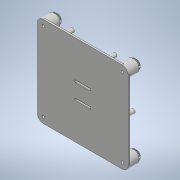
# Autodesk Inventor part: Зажим проводов
Saved by Autodesk Inventor 2020 (Build 240168000, 168)
## iProperties
Created: 2021-04-22
Part Number: Зажим проводов
Material: Типовые
Document SubType Name: Modeling
Designer: I_Love_U_Bogdan
Density: 1 g/cm^3
Appearance: По умолчанию
Author: I_Love_U_Bogdan
Autodesk Inventor part; units mm, degrees
ref_plane "YZ Plane" through (0, 0, 0) normal (1, 0, 0) x (0, 1, 0)
ref_plane "XZ Plane" through (0, 0, 0) normal (0, 1, 0) x (-1, 0, 0)
ref_plane "XY Plane" through (0, 0, 0) normal (0, 0, 1) x (1, 0, 0)
sketch "Эскиз1" plane through (0, 0, 0) normal (0, 0, 1) x (1, 0, 0)
  circle A0 centre (-37.4959, 38.6601) radius 4.5 projected
  circle A1 centre (62.5041, 38.6601) radius 4.5 projected
  line L0 (-47.4959, 36.6601) -> (-44.978, 39.178) projected
  line L1 (-47.4959, 36.6601) -> (-47.4959, -61.7399) projected
  line L2 (-40.4959, -68.7399) -> (-47.4959, -61.7399) projected
  line L3 (-40.4959, -68.7399) -> (65.5041, -68.7399) projected
  line L4 (72.5041, -61.7399) -> (65.5041, -68.7399) projected
  line L5 (72.5041, -61.7399) -> (72.5041, 36.6601) projected
  line L6 (69.9862, 39.178) -> (72.5041, 36.6601) projected
  arc A2 (69.9862, 39.178) -> (56.914, 43.6601) centre (62.5041, 38.6601) ccw projected
  line L7 (56.914, 43.6601) -> (-31.9057, 43.6601) projected
  arc A3 (-31.9057, 43.6601) -> (-44.978, 39.178) centre (-37.4959, 38.6601) ccw projected
  circle A4 centre (-37.4959, -60.7399) radius 4.5 projected
  circle A5 centre (62.5041, -60.7399) radius 4.5 projected
  circle A6 centre (7.5041, -49.0399) radius 2.5 projected
  circle A7 centre (31.8041, -37.6685) radius 2.5 projected
  circle A8 centre (16.6041, 13.1315) radius 2.5 projected
  circle A9 centre (-41.4959, 8.9601) radius 2.5 projected
  circle A10 centre (7.5041, 8.9601) radius 2.5 projected
  circle A11 centre (64.8041, 14.4315) radius 2.5 projected
  circle A12 centre (59.7041, -37.6685) radius 2.5 projected
  circle A13 centre (-41.4959, -49.0399) radius 2.5 projected
  circle A14 centre (-37.4959, 38.6601) radius 7.5
  circle A15 centre (62.5041, 38.6601) radius 7.5
  circle A16 centre (62.5041, -60.7399) radius 7.5
  circle A17 centre (-37.4959, -60.7399) radius 7.5
  circle A18 centre (39.5041, 38.6601) radius 2.5
  circle A19 centre (-14.4959, 38.6601) radius 2.5
  circle A20 centre (-14.4959, 13.6601) radius 2.5
  circle A21 centre (39.5041, 13.6601) radius 2.5
  circle A22 centre (-14.4959, -11.3399) radius 2.5
  circle A23 centre (39.5041, -11.3399) radius 2.5
  circle A24 centre (-14.4959, -36.3399) radius 2.5
  circle A25 centre (39.5041, -36.3399) radius 2.5
  circle A26 centre (-14.4959, -61.3399) radius 2.5
  circle A27 centre (39.5041, -61.3399) radius 2.5
  circle A28 centre (62.5041, -11.3399) radius 2.5
  circle A29 centre (-37.4959, -11.3399) radius 2.5
  point P0 (0, 0)
  dimension "d0" = 3
  dimension "d1" = 3
  dimension "d2" = 3
  dimension "d3" = 3
  dimension "d4" = 5
  dimension "d5" = 5
  dimension "d6" = 23
  dimension "d7" = 23
  dimension "d8" = 5
  dimension "d9" = 5
  dimension "d12" = 25
  dimension "d17" = 5
  dimension "d18" = 5
  dimension "d19" = 0
  dimension "d20" = 50
  dimension "d21" = 50
  constraints: 16 centre point, 1 vertical, 16 other
  measures "d0" radial gap between concentric circles of A0 A14
  measures "d1" radial gap between concentric circles of A1 A15
  measures "d2" radial gap between concentric circles of A5 A16
  measures "d3" radial gap between concentric circles of A4 A17
  measures "d4" diameter of A18
  measures "d5" diameter of A19
  measures "d6" distance of A19.centre A0.centre
  measures "d7" distance of A1.centre A18.centre
  measures "d8" distance from line of L7 A18.centre
  measures "d9" distance from line of L7 A19.centre
  measures "d12" distance of A19.centre A20.centre
  measures "d17" diameter of A28
  measures "d18" diameter of A29
  measures "d19" horizontal distance of A29.centre A4.centre
  measures "d20" vertical distance of A28.centre A18.centre
  measures "d21" vertical distance of A19.centre A29.centre
extrude "Выдавливание1" add sketch "Эскиз1" along normal blind 12 contours A0 | A1 | A3 A14 | A2 A15 | A4 | A5 | A16 | A17 | A18 | A19 | A20 | A21 | A22 | A23 | A24 | A25 | A26 | A27 | A28 | A29
sketch "Эскиз2" plane through (-37.4959, -60.7399, 12) normal (0, 0, 1) x (1, 0, 0)
  circle A0 centre (0, 0) radius 7.5 projected
  circle A1 centre (100, 0) radius 7.5 projected
  circle A2 centre (100, 99.4) radius 7.5 projected
  circle A3 centre (0, 99.4) radius 7.5 projected
  circle A4 centre (0, 0) radius 7.5 projected
  line L0 (0, -7.5) -> (100, -7.5)
  circle A5 centre (100, 0) radius 7.5 projected
  line L1 (107.5, 0) -> (107.5, 99.4)
  circle A6 centre (100, 99.4) radius 7.5 projected
  line L2 (100, 106.9) -> (0, 106.9)
  circle A7 centre (0, 99.4) radius 7.5 projected
  line L3 (-7.5, 99.4) -> (-7.5, 0)
  point P0 (37.4959, 60.7399)
  point P1 (-7.5, 99.4)
  point P2 (0, -7.5)
  point P3 (100, -7.5)
  constraints: 8 end point, 3 horizontal, 3 vertical, 2 vertical alignment, 1 horizontal alignment, 1 perpendicular, 1 point on circle, 1 tangent, 11 other
extrude "Выдавливание2" add sketch "Эскиз2" along normal blind 2
sketch "Эскиз3" plane through (-37.4959, 38.6601, 0) normal (0, 0, -1) x (-1, 0, 0)
  circle A0 centre (-100, 0) radius 4.5 projected
  circle A1 centre (-100, -99.4) radius 4.5 projected
  circle A2 centre (0, -99.4) radius 4.5 projected
  circle A3 centre (0, 0) radius 4.5 projected
  circle A4 centre (0, 0) radius 4.3
  circle A5 centre (-100, 0) radius 4.3
  circle A6 centre (-100, -99.4) radius 4.3
  circle A7 centre (0, -99.4) radius 4.3
  point P0 (-37.4959, -38.6601)
  dimension "d26" = 0.2
  dimension "d27" = 0.2
  dimension "d28" = 0.2
  dimension "d29" = 0.2
  constraints: 4 centre point
  measures "d26" radial gap between concentric circles of A3 A4
  measures "d27" radial gap between concentric circles of A0 A5
  measures "d28" radial gap between concentric circles of A1 A6
  measures "d29" radial gap between concentric circles of A2 A7
extrude "Выдавливание3" add sketch "Эскиз3" along normal blind 2.2 contours A4 | A5 | A6 | A7
sketch "Эскиз4" plane through (-37.4959, 38.6601, -2.2) normal (0, 0, -1) x (-1, 0, 0)
  circle A0 centre (0, 0) radius 4.3 projected
  circle A1 centre (-100, 0) radius 4.3 projected
  circle A2 centre (-100, -99.4) radius 4.3 projected
  circle A3 centre (0, -99.4) radius 4.3 projected
  circle A4 centre (0, 0) radius 6.3
  circle A5 centre (-100, 0) radius 6.3
  circle A6 centre (-100, -99.4) radius 6.3
  circle A7 centre (0, -99.4) radius 6.3
  point P0 (-37.4959, -38.6601)
  dimension "d32" = 2
  dimension "d33" = 2
  dimension "d34" = 2
  dimension "d35" = 2
  constraints: 4 centre point, 1 coincident
  measures "d32" radial gap between concentric circles of A4 A0
  measures "d33" radial gap between concentric circles of A1 A5
  measures "d34" radial gap between concentric circles of A2 A6
  measures "d35" radial gap between concentric circles of A3 A7
extrude "Выдавливание4" add sketch "Эскиз4" along normal blind 2.2 contours A0 | A1 | A2 | A3 | A4 | A5 | A6 | A7
chamfer "Фаска1" distance 2 angle 45 4 edges at (-31.1959, 38.6601, -4.4) (68.8041, 38.6601, -4.4) (68.8041, -60.7399, -4.4) (-31.1959, -60.7399, -4.4)
sketch "Эскиз5" plane through (62.5041, 38.6601, -4.4) normal (0, 0, -1) x (-1, 0, 0)
  circle A0 centre (100, 0) radius 4.3 projected
  circle A1 centre (0, 0) radius 4.3 projected
  circle A2 centre (0, -99.4) radius 4.3 projected
  circle A3 centre (100, -99.4) radius 4.3 projected
  line L0 (101, 10) -> (99, 10)
  line L1 (99, 10) -> (99, -10)
  line L2 (99, -10) -> (101, -10)
  line L3 (101, -10) -> (101, 10)
  line L4 (101, 10) -> (99, -10) construction
  line L5 (99, 10) -> (101, -10) construction
  line L6 (110, 1) -> (90, 1)
  line L7 (90, 1) -> (90, -1)
  line L8 (90, -1) -> (110, -1)
  line L9 (110, -1) -> (110, 1)
  line L10 (110, 1) -> (90, -1) construction
  line L11 (90, 1) -> (110, -1) construction
  arc A4 (-7.5, 0) -> (0, 7.5) centre (0, 0) ccw projected
  line L12 (-7.5, -99.4) -> (-7.5, 0) projected
  arc A5 (0, -106.9) -> (-7.5, -99.4) centre (0, -99.4) ccw projected
  line L13 (100, -106.9) -> (0, -106.9) projected
  arc A6 (107.5, -99.4) -> (100, -106.9) centre (100, -99.4) ccw projected
  line L14 (107.5, 0) -> (107.5, -99.4) projected
  arc A7 (100, 7.5) -> (107.5, 0) centre (100, 0) ccw projected
  line L15 (0, 7.5) -> (100, 7.5) projected
  circle A8 centre (77, -100) radius 2.5 projected
  circle A9 centre (23, -50) radius 2.5 projected
  circle A10 centre (77, -75) radius 2.5 projected
  circle A11 centre (77, -50) radius 2.5 projected
  circle A12 centre (23, 0) radius 2.5 projected
  circle A13 centre (0, -50) radius 2.5 projected
  circle A14 centre (23, -100) radius 2.5 projected
  circle A15 centre (23, -75) radius 2.5 projected
  circle A16 centre (77, 0) radius 2.5 projected
  circle A17 centre (77, -25) radius 2.5 projected
  circle A18 centre (23, -25) radius 2.5 projected
  circle A19 centre (100, -50) radius 2.5 projected
  line L16 (99, -89.4) -> (101, -89.4)
  line L17 (101, -89.4) -> (101, -109.4)
  line L18 (101, -109.4) -> (99, -109.4)
  line L19 (99, -109.4) -> (99, -89.4)
  line L20 (99, -89.4) -> (101, -109.4) construction
  line L21 (101, -89.4) -> (99, -109.4) construction
  line L22 (110, -98.4) -> (90, -98.4)
  line L23 (90, -98.4) -> (90, -100.4)
  line L24 (90, -100.4) -> (110, -100.4)
  line L25 (110, -100.4) -> (110, -98.4)
  line L26 (110, -98.4) -> (90, -100.4) construction
  line L27 (90, -98.4) -> (110, -100.4) construction
  line L28 (-1, -89.4) -> (1, -89.4)
  line L29 (10, -98.4) -> (-10, -98.4)
  line L30 (-10, -98.4) -> (-10, -100.4)
  line L31 (-10, -100.4) -> (10, -100.4)
  line L32 (10, -98.4) -> (-10, -100.4) construction
  line L33 (-10, -98.4) -> (10, -100.4) construction
  line L34 (10, -100.4) -> (10, -98.4)
  line L35 (1, -89.4) -> (1, -109.4)
  line L36 (-1, -89.4) -> (1, -109.4) construction
  line L37 (1, -89.4) -> (-1, -109.4) construction
  line L38 (1, -109.4) -> (-1, -109.4)
  line L39 (-1, -109.4) -> (-1, -89.4)
  line L40 (-1, -10) -> (1, -10)
  line L41 (-10, 1) -> (-10, -1)
  line L42 (10, 1) -> (-10, 1)
  line L43 (-10, -1) -> (10, -1)
  line L44 (10, 1) -> (-10, -1) construction
  line L45 (-10, 1) -> (10, -1) construction
  line L46 (10, -1) -> (10, 1)
  line L47 (1, 10) -> (-1, 10)
  line L48 (1, -10) -> (1, 10)
  line L49 (1, 10) -> (-1, -10) construction
  line L50 (-1, 10) -> (1, -10) construction
  line L51 (-1, 10) -> (-1, -10)
  point P0 (62.5041, -38.6601)
  point P1 (0, -99.4)
  point P2 (0, 0)
  point P3 (1, 1)
  point P4 (-1, 1)
  point P5 (-1, -1)
  point P6 (1, -1)
  point P7 (-1, -98.4)
  point P8 (-1, -100.4)
  point P9 (1, -100.4)
  point P10 (1, -98.4)
  point P11 (99, -100.4)
  point P12 (101, -100.4)
  point P13 (101, -98.4)
  point P14 (99, -98.4)
  point P15 (101, -1)
  point P16 (101, 1)
  point P17 (99, 1)
  point P18 (99, -1)
  dimension "d41" = 2
  dimension "d42" = 20
  dimension "d43" = 20
  dimension "d44" = 2
  dimension "d45" = 2
  dimension "d46" = 20
  dimension "d47" = 20
  dimension "d48" = 2
  dimension "d51" = 100
  constraints: 96 end point, 16 midpoint, 8 parallel, 5 horizontal, 4 perpendicular, 42 other
  measures "d41" distance of L2.end L1.end
  measures "d42" distance of L1.end L0.end
  measures "d43" distance of L8.end L7.end
  measures "d44" distance of L7.end L6.end
  measures "d45" distance of L17.end L18.end
  measures "d46" distance of L16.end L17.end
  measures "d47" distance of L24.end L23.end
  measures "d48" distance of L23.end L22.end
  measures "d51" distance of L16.start L28.start
extrude "Выдавливание5" cut sketch "Эскиз5" against normal blind 5 contours A0 L8 L3 L6 | A0 L6 L9 L8 L14 A7 | L3 L6 L1 A0 | A0 L1 A7 L15 L0 L3 | L3 L8 L1 L6 | L3 A7 L1 A0 | A0 L1 L8 L3 | A7 L14 L8 | L1 L8 A0 L6 | L3 L2 L1 A7 | A0 L8 A7 L6 | L1 L15 A7 | L22 L25 L24 A3 A6 L14 | L14 A6 L22 | A7 L8 L7 L6 | L48 A4 L15 | L15 A4 L48 A1 L51 L47 | L17 A3 L19 A6 | A6 L19 L16 L17 | A3 L24 L17 L22 | L17 L22 L19 A3 | L17 L24 L19 L22 | L42 L46 L43 A4 | A4 L43 A1 L42 | L48 L42 L51 A1 | L17 L18 L19 L13 A6 A3 | A3 L19 L24 L17 | L22 A3 L24 A6 | A6 L24 L23 L22 | L19 L24 A3 L22 | A1 L43 L48 L42 | L48 L43 L51 L42 | L48 L40 L51 A4 | A4 L51 A1 L48 | L42 L51 L43 A1 | A1 L43 A4 L12 L41 L42 | L48 A1 L51 L43 | A6 L13 L19 | L43 L12 A4 | L35 L38 L39 A2 A5 L13 | L13 A5 L35 | L29 A5 L12 | L12 A5 L29 A2 L31 L30 | L31 A2 L29 A5 | A5 L29 L34 L31 | A2 L39 L31 L35 | L31 L35 L29 A2 | L31 L39 L29 L35 | L39 L28 L35 A5 | A5 L35 A2 L39 | L29 L39 L31 A2 | L29 L39 A2 L35
sketch "Эскиз6" plane through (-37.4959, -60.7399, 14) normal (0, 0, 1) x (1, 0, 0)
  arc A0 (107.5, 99.4) -> (100, 106.9) centre (100, 99.4) ccw projected
  arc A1 (100, -7.5) -> (107.5, 0) centre (100, 0) ccw projected
  arc A2 (0, 106.9) -> (-7.5, 99.4) centre (0, 99.4) ccw projected
  arc A3 (-7.5, 0) -> (0, -7.5) centre (0, 0) ccw projected
  circle A4 centre (0, 0) radius 1.5
  circle A5 centre (0, 99.4) radius 1.5
  circle A6 centre (100, 99.4) radius 1.5
  circle A7 centre (100, 0) radius 1.5
  circle A8 centre (77, 49.4) radius 2.5 projected
  circle A9 centre (23, 49.4) radius 2.5 projected
  line L0 (77, 49.4) -> (23, 49.4)
  line L1 (50, 49.4) -> (50, 39.4)
  line L2 (50, 49.4) -> (50, 59.4)
  line L3 (40, 60.4) -> (60, 60.4)
  line L4 (60, 60.4) -> (60, 58.4)
  line L5 (60, 58.4) -> (40, 58.4)
  line L6 (40, 58.4) -> (40, 60.4)
  line L7 (40, 60.4) -> (60, 58.4) construction
  line L8 (60, 60.4) -> (40, 58.4) construction
  line L9 (40, 40.4) -> (60, 40.4)
  line L10 (60, 40.4) -> (60, 38.4)
  line L11 (60, 38.4) -> (40, 38.4)
  line L12 (40, 38.4) -> (40, 40.4)
  line L13 (40, 40.4) -> (60, 38.4) construction
  line L14 (60, 40.4) -> (40, 38.4) construction
  point P0 (37.4959, 60.7399)
  dimension "d58" = 3
  dimension "d59" = 3
  dimension "d60" = 3
  dimension "d61" = 3
  dimension "d64" = 10
  dimension "d65" = 10
  dimension "d66" = 20
  dimension "d67" = 2
  dimension "d68" = 20
  dimension "d69" = 2
  constraints: 30 end point, 5 midpoint, 4 centre point, 4 coincident, 4 parallel, 3 horizontal, 2 perpendicular, 2 vertical
  measures "d58" diameter of A4
  measures "d59" diameter of A5
  measures "d60" diameter of A6
  measures "d61" diameter of A7
  measures "d64" distance of L1.start L1.end
  measures "d65" distance of L1.start L2.end
  measures "d66" distance of L4.end L5.end
  measures "d67" distance of L3.end L4.end
  measures "d68" distance of L10.end L11.end
  measures "d69" distance of L9.end L10.end
extrude "Выдавливание6" cut sketch "Эскиз6" against normal blind 5 contours A4 | A5 | A6 | A7 | L3 L4 L5 L6 | L9 L10 L11 L12
fillet "Сопряжение1" radius 1 8 edges at (2.5041, -0.3399, 13) (2.5041, -2.3399, 13) (22.5041, -2.3399, 13) (22.5041, -0.3399, 13) (2.5041, -22.3399, 13) (2.5041, -20.3399, 13) (22.5041, -22.3399, 13) (22.5041, -20.3399, 13)
chamfer "Фаска2" distance 0.5 angle 45 4 edges at (12.5041, -22.3399, 14) (12.5041, -20.3399, 14) (12.5041, -2.3399, 14) (12.5041, -0.3399, 14)
